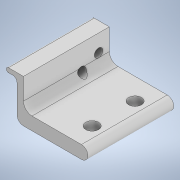
# Autodesk Inventor part: Cable_Guide_Support_small
Saved by Autodesk Inventor 2021 (Build 250183000, 183)
## iProperties
Created: 2022-01-07
Part Number: Cable_Guide_Support_small
Material: Generic
Document SubType Name: Modeling
Designer: Jorian Brusind
Density: 1 g/cm^3
Appearance: Default
Author: Jorian Brusind
Autodesk Inventor part; units mm, degrees
ref_plane "YZ Plane" through (0, 0, 0) normal (1, 0, 0) x (0, 1, 0)
ref_plane "XZ Plane" through (0, 0, 0) normal (0, 1, 0) x (-1, 0, 0)
ref_plane "XY Plane" through (0, 0, 0) normal (0, 0, 1) x (1, 0, 0)
sketch "Sketch1" plane through (0, 0, 0) normal (0, 1, 0) x (-1, 0, 0)
  line L0 (0, 0) -> (33, 0)
  line L1 (33, 0) -> (33, -40)
  line L2 (33, -40) -> (0, -40)
  line L3 (0, -40) -> (0, 0)
  dimension "d0" = 33
  dimension "d1" = 40
  constraints: 8 end point, 2 parallel, 1 horizontal, 1 perpendicular
  measures "d0" distance of L1.end L2.end
  measures "d1" distance of L0.end L1.end
extrude "Extrusion1" add sketch "Sketch1" along normal blind 6
sketch "Sketch2" plane through (0, 6, 0) normal (0, 1, 0) x (1, 0, 0)
  line L0 (-33, 0) -> (0, 0) projected
  line L1 (0, 40) -> (-33, 40) projected
  line L2 (-33, 0) -> (-30, 0)
  line L3 (-30, 0) -> (-30, 40)
  line L4 (-30, 40) -> (-33, 40)
  line L5 (-33, 40) -> (-33, 0)
  dimension "d4" = 3
  constraints: 8 end point, 2 parallel, 1 horizontal, 1 perpendicular, 1 point on line
  measures "d4" distance of L4.end L3.end
extrude "Extrusion2" add sketch "Sketch2" along normal blind 14
sketch "Sketch3" plane through (-33, 0, -40) normal (-1, 0, 0) x (0, 0, 1)
  line L0 (0, 20) -> (40, 20) projected
  line L1 (40, 20) -> (0, 20)
  line L2 (0, 20) -> (0, 18)
  line L3 (0, 18) -> (40, 18)
  line L4 (40, 18) -> (40, 20)
  point P0 (40, 0)
  point P1 (0, 20)
  dimension "d7" = 40
  dimension "d8" = 2
  constraints: 8 end point, 2 parallel, 1 horizontal, 1 perpendicular
  measures "d7" distance of L3.end L2.end
  measures "d8" distance of L2.end L1.end
extrude "Extrusion3" add sketch "Sketch3" along normal blind 5
fillet "Fillet1" radius 1 2 edges at (-38, 20, -20) (-38, 18, -20)
fillet "Fillet2" radius 4 1 edges at (-30, 6, -20)
fillet "Fillet3" radius 3 2 edges at (0, 6, -20) (0, 0, -20)
fillet "Fillet4" radius 3 1 edges at (-33, 0, -20)
sketch "Sketch4" plane through (0, 6, 0) normal (0, 1, 0) x (1, 0, 0)
  line L0 (-8, 0) -> (-8, 10)
  line L1 (-3, 40) -> (-30, 40) projected
  circle A0 centre (-8, 10) radius 3
  line L2 (-8, 40) -> (-8, 30)
  line L3 (-8, 40) -> (2, 40) construction
  circle A1 centre (-8, 30) radius 3
  point P0 (0, 0)
  dimension "d15" = 10
  dimension "d16" = 6
  dimension "d17" = 10
  dimension "d18" = 90
  dimension "d19" = 5
  dimension "d20" = 6
  dimension "d23" = 5
  constraints: 6 end point, 2 centre point, 2 coincident, 2 perpendicular, 1 horizontal, 1 point on line, 1 vertical
  measures "d15" distance of L0.start L0.end
  measures "d16" diameter of A0
  measures "d17" distance of L2.start L2.end
  measures "d18" angle of L2 L3
  measures "d19" distance from line of L1.start L2
  measures "d20" diameter of A1
  measures "d23" distance from line of L1.start L0
extrude "Extrusion4" cut sketch "Sketch4" against normal through all
fillet "Fillet5" radius 2 1 edges at (-33, 18, -20)
sketch "Sketch5" plane through (-33, 3, -40) normal (-1, 0, 0) x (0, 0, 1)
  line L0 (0, 5.5) -> (5, 5.5)
  line L1 (5, 5.5) -> (5, 9)
  line L2 (5, 5.5) -> (8.5, 5.5) construction
  line L3 (5, 5.5) -> (13, 5.5)
  circle A0 centre (5, 9) radius 2
  circle A1 centre (13, 5.5) radius 2
  line L4 (40, 0) -> (0, 0) projected
  line L5 (0, 7) -> (0, 17) projected
  line L6 (0, -3) -> (40, -3) projected
  dimension "d25" = 5
  dimension "d28" = 3.5
  dimension "d29" = 90
  dimension "d30" = 8
  dimension "d32" = 4
  dimension "d33" = 4
  dimension "d38" = 8.5
  constraints: 8 end point, 2 centre point, 2 coincident, 2 horizontal, 1 perpendicular, 1 point on line, 1 vertical
  measures "d25" distance of L0.start L0.end
  measures "d28" distance of L0.end L1.end
  measures "d29" angle of L2 L1
  measures "d30" distance of L0.end L3.end
  measures "d32" diameter of A0
  measures "d33" diameter of A1
  measures "d38" distance between parallel lines of L6 L0
extrude "Extrusion5" cut sketch "Sketch5" against normal through all both and the other way through all
body "Solid1"
